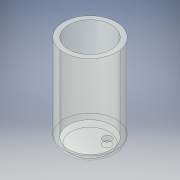
# Autodesk Inventor part: bottun tube
Saved by Autodesk Inventor 2018 (Build 220112000, 112)
## iProperties
Created: 2018-02-28
Part Number: bottun tube
Material: Glass
Document SubType Name: Modeling
Designer: 238438
Density: 2.18 g/cm^3
Appearance: Clear
Author: 238438
Autodesk Inventor part; units mm, degrees
ref_plane "YZ Plane" through (0, 0, 0) normal (1, 0, 0) x (0, 1, 0)
ref_plane "XZ Plane" through (0, 0, 0) normal (0, 1, 0) x (-1, 0, 0)
ref_plane "XY Plane" through (0, 0, 0) normal (0, 0, 1) x (1, 0, 0)
sketch "Sketch1" plane through (0, 0, 0) normal (0, 1, 0) x (-1, 0, 0)
  circle A0 centre (0, 0) radius 5.842
  dimension "d0" = 11.684
  constraints: 1 centre point, 1 coincident
  measures "d0" diameter of A0
extrude "Extrusion1" add sketch "Sketch1" along normal blind 20.32
shell "Shell1" thickness 1.0922 removed faces 1 at (-0.5241, 20.32, 1.3818)
fillet "Fillet1" radius 1.5875 1 edges at (5.842, 0, 0)
sketch "Sketch2" plane through (0, 0, 0) normal (0, -1, 0) x (1, 0, 0)
  circle A0 centre (2.1901, -1.6223) radius 0.9525
  point P0 (0, 0)
  dimension "d5" = 1.905
  constraints: 1 centre point
  measures "d5" diameter of A0
extrude "Extrusion2" cut sketch "Sketch2" against normal through all
body "Solid1"
